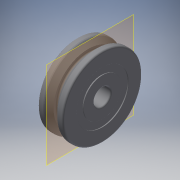
# Autodesk Inventor part: W2RX Bearing
Saved by Autodesk Inventor 2018.3 (Build 223284000, 284)
## iProperties
Category: PARTsolutions
Company: BWC
Created: 2020-02-15
Part Number: W2RX Bearing
Material: Generic
Catalog Web Link: www.cadenas.de
Description: Radial Wheels-Radial Wheels
Vendor: BWC
Document SubType Name: Modeling
Designer: psadmin
Manufacturer: BWC
Mass: 5.93829 g
Surface Area: 30.052 cm^2
Volume: 5.93829 cm^3
Density: 1 g/cm^3
Appearance: PSOLRGB-175-175-175
PSOL_IDENT_0: {$CADENAS_DATA\23d-libs\bwc\madewell\radial_wheels.prj},158 {VTYP=3D},{NB=W2RX},{LINA=W2RX},{NN=Radi
PSOL_IDENT_1: al Wheels},{DATE=05.12.2019 09:46:06},{GEOMDATE=08.11.2014 11:33:08},{VERSION=},{LINEID=30},{WBVAR=M
PSOL_IDENT_2: AT},{WBNUMERIC=}  {NB=W2RX},{LINA=W2RX},{KT=DUMMY},{PN=W2RX},{MAT=RX},{SIZE=2},{D=1.210},{W=0.3830},
PSOL_IDENT_3: {B=0.2510},{VRI=0.5000},{C=0.020},{C1=0.584},{E=0.024},{R=0.028},{R1=0.008},{A=1.3018},{F=0.1250},{R
PSOL_IDENT_4: LN=1500},{RLLBF=337},{ALN=320},{ALLBF=72},{CATEGALG=Radial Wheel, Size 2, Carbon Steel, Sealed},{FEA
PSOL_IDENT_5: TALG=<li style=\" margin-top:0px; margin-bottom:0px; margin-left:0px; margin-right:0px; -qt-block-in
PSOL_IDENT_6: dent:0; text-indent:0px;\"><span style=\" font-size:11pt; font-weight:600;\">General purpose AISI 52
PSOL_IDENT_7: 100 carbon steel</span></li><li style=\" font-size:11pt; font-weight:600;\" style=\" margin-top:0px;
PSOL_IDENT_8: margin-bottom:0px; margin-left:0px; margin-right:0px; -qt-block-indent:0; text-indent:0px;\">Single
PSOL_IDENT_9: row deep-groove ball bearing</li><li style=\" font-size:11pt; font-weight:600;\" style=\" margin-to
PSOL_IDENT_10: p:0px; margin-bottom:0px; margin-left:0px; margin-right:0px; -qt-block-indent:0; text-indent:0px;\">
PSOL_IDENT_11: Precision ground 90° vee inside running surfaces</li><li style=\" font-size:11pt; font-weight:600;\"
PSOL_IDENT_12: style=\" margin-top:0px; margin-bottom:0px; margin-left:0px; margin-right:0px; -qt-block-indent:0;
PSOL_IDENT_13: text-indent:0px;\">Hardened for heavy loads and durability</li><li style=\" font-size:11pt; font-wei
PSOL_IDENT_14: ght:600;\" style=\" margin-top:0px; margin-bottom:0px; margin-left:0px; margin-right:0px; -qt-block-
PSOL_IDENT_15: indent:0; text-indent:0px;\">Seals to protect against contamination</li>},{DESCRALG=<span style=\" f
PSOL_IDENT_16: ont-size:11pt; font-weight:600;\">MadeWell radial wheels are linear guide bearings with single row d
PSOL_IDENT_17: eep-groove ball arrangement with precision ground 90° vee inside surfaces to support loads and provi
PSOL_IDENT_18: de smooth and quiet motion. They are an ideal choice for low cost linear guide bearings in simple li
PSOL_IDENT_19: near guide applications such as doors and windows, museum displays, cabinets, and automation.  Use w
PSOL_IDENT_20: ith DualVee guide track for linear motion. General purpose carbon steel with rubber seals protect ag
PSOL_IDENT_21: ainst small particle contamination. Through bore allows mounting with common bolts and washers. Inte
PSOL_IDENT_22: rnically lubricated for life with general purpose grease.</span>},{RATINGSALG=<span style=\" font-si
PSOL_IDENT_23: ze:11pt; font-weight:600; color:#000000;\">Temperature Range:</span><span style=\" font-size:11pt; c
PSOL_IDENT_24: olor:#000000;\"> -20°C to +100°C</span></p><p style=\" margin-top:0px; margin-bottom:0px; margin-lef
PSOL_IDENT_25: t:0px; margin-right:0px; -qt-block-indent:0; text-indent:0px;\"><span style=\" font-size:11pt; font-
PSOL_IDENT_26: weight:600; color:#000000;\">RoHS Compliant</span>}
NN: Radial Wheels
NT: Radial Wheels
NB: W2RX
NBSYN: $PN.
LINA: W2RX
PN: W2RX
MAT: AISI 52100 Carbon steel
SIZE: 2
D: 1.21
W: 0.383
B: 0.251
VRI: 0.5
RLN: 1500
RLLBF: 337
ALN: 320
ALLBF: 72
SUPPLIER: BWC
ARTICLENO: W2RX
BOMINFO: W2RX
CREATOR: CADENAS GmbH
Title: W2RX
Author: Cadenas PARTsolutions
Comments: Radial Wheels
Autodesk Inventor part; units mm, degrees
sketch "Sketch_1" plane through (0, 0, 0) normal (0, 0, 1) x (1, 0, 0)
  line L0 (4.8641, 0) -> (-4.8641, 0)
  line L1 (-4.8641, 7.3152) -> (-4.8641, 3.6957)
  arc A0 (-4.8641, 3.6957) -> (-4.3561, 3.1877) centre (-4.3561, 3.6957) ccw
  line L2 (-4.3561, 3.1877) -> (4.3561, 3.1877)
  arc A1 (4.3561, 3.1877) -> (4.8641, 3.6957) centre (4.3561, 3.6957) ccw
  line L3 (4.8641, 3.6957) -> (4.8641, 7.3152)
  arc A2 (4.8641, 7.3152) -> (4.7625, 7.4168) centre (4.7625, 7.3152) ccw
  line L4 (4.7625, 7.4168) -> (4.6609, 7.4168)
  arc A3 (4.6609, 7.4168) -> (4.5593, 7.3152) centre (4.6609, 7.3152) ccw
  line L5 (4.5593, 7.3152) -> (4.5593, 7.112)
  line L6 (4.5593, 7.112) -> (4.2545, 7.112)
  line L7 (4.2545, 7.112) -> (4.2545, 10.2616)
  arc A4 (4.3561, 10.3632) -> (4.2545, 10.2616) centre (4.3561, 10.2616) ccw
  line L8 (4.3561, 10.3632) -> (4.5593, 10.3632)
  line L9 (4.5593, 10.3632) -> (4.5593, 10.16)
  arc A5 (4.5593, 10.16) -> (4.6609, 10.0584) centre (4.6609, 10.16) ccw
  line L10 (4.6609, 10.0584) -> (4.7625, 10.0584)
  arc A6 (4.7625, 10.0584) -> (4.8641, 10.16) centre (4.7625, 10.16) ccw
  line L11 (4.8641, 10.16) -> (4.8641, 14.7574)
  arc A7 (4.8641, 14.7574) -> (4.2545, 15.367) centre (4.2545, 14.7574) ccw
  line L12 (4.2545, 15.367) -> (2.8699, 15.367)
  line L13 (2.8699, 15.367) -> (2.523, 15.2233)
  line L14 (2.523, 15.2233) -> (0.7112, 13.4115)
  line L15 (0.7112, 13.4115) -> (0.7112, 12.7)
  arc A8 (-0.7112, 12.7) -> (0.7112, 12.7) centre (0, 12.7) ccw
  line L16 (-0.7112, 12.7) -> (-0.7112, 13.4115)
  line L17 (-0.7112, 13.4115) -> (-2.523, 15.2233)
  line L18 (-2.523, 15.2233) -> (-2.8699, 15.367)
  line L19 (-2.8699, 15.367) -> (-4.2545, 15.367)
  arc A9 (-4.2545, 15.367) -> (-4.8641, 14.7574) centre (-4.2545, 14.7574) ccw
  line L20 (-4.8641, 14.7574) -> (-4.8641, 10.16)
  arc A10 (-4.8641, 10.16) -> (-4.7625, 10.0584) centre (-4.7625, 10.16) ccw
  line L21 (-4.7625, 10.0584) -> (-4.6609, 10.0584)
  arc A11 (-4.6609, 10.0584) -> (-4.5593, 10.16) centre (-4.6609, 10.16) ccw
  line L22 (-4.5593, 10.16) -> (-4.5593, 10.3632)
  line L23 (-4.5593, 10.3632) -> (-4.3561, 10.3632)
  arc A12 (-4.2545, 10.2616) -> (-4.3561, 10.3632) centre (-4.3561, 10.2616) ccw
  line L24 (-4.2545, 10.2616) -> (-4.2545, 7.112)
  line L25 (-4.2545, 7.112) -> (-4.5593, 7.112)
  line L26 (-4.5593, 7.112) -> (-4.5593, 7.3152)
  arc A13 (-4.5593, 7.3152) -> (-4.6609, 7.4168) centre (-4.6609, 7.3152) ccw
  line L27 (-4.6609, 7.4168) -> (-4.7625, 7.4168)
  arc A14 (-4.7625, 7.4168) -> (-4.8641, 7.3152) centre (-4.7625, 7.3152) ccw
  constraints: 56 end point, 30 point on circle, 15 centre point
revolve "Revolution1" add sketch "Sketch_1" angle 360 about axis through (4.8641, 0, 0) along (1, 0, 0)
ref_plane "b_XY" through (-4.6609, 3.1877, 0) normal (0, 0, 1) x (1, 0, 0)
ref_plane "b_YZ" through (-4.6609, 3.1877, 0) normal (1, 0, 0) x (0, 1, 0)
ref_plane "b_ZX" through (-4.6609, 3.1877, 0) normal (0, 1, 0) x (0, 0, 1)
ref_plane "b1_XY" through (-4.6609, -3.1877, 0) normal (0, 0, 1) x (1, 0, 0)
ref_plane "b1_YZ" through (-4.6609, -3.1877, 0) normal (1, 0, 0) x (0, 1, 0)
ref_plane "b1_ZX" through (-4.6609, -3.1877, 0) normal (0, 1, 0) x (0, 0, 1)
ref_plane "d_XY" through (-2.4321, 15.367, 0) normal (0, 0, 1) x (1, 0, 0)
ref_plane "d_YZ" through (-2.4321, 15.367, 0) normal (1, 0, 0) x (0, 1, 0)
ref_plane "d_ZX" through (-2.4321, 15.367, 0) normal (0, 1, 0) x (0, 0, 1)
ref_plane "d1_XY" through (-2.4321, -15.367, 0) normal (0, 0, 1) x (1, 0, 0)
ref_plane "d1_YZ" through (-2.4321, -15.367, 0) normal (1, 0, 0) x (0, 1, 0)
ref_plane "d1_ZX" through (-2.4321, -15.367, 0) normal (0, 1, 0) x (0, 0, 1)
ref_plane "vri_XY" through (0, 12.7, 0) normal (0, 0, 1) x (1, 0, 0)
ref_plane "vri_YZ" through (0, 12.7, 0) normal (1, 0, 0) x (0, 1, 0)
ref_plane "vri_ZX" through (0, 12.7, 0) normal (0, 1, 0) x (0, 0, 1)
ref_plane "vri1_XY" through (4.8641, 0, 0) normal (0, 0, 1) x (1, 0, 0)
ref_plane "vri1_YZ" through (4.8641, 0, 0) normal (1, 0, 0) x (0, 1, 0)
ref_plane "vri1_ZX" through (4.8641, 0, 0) normal (0, 1, 0) x (0, 0, 1)
ref_plane "w_XY" through (-4.8641, 12.7, 0) normal (0, 0, 1) x (1, 0, 0)
ref_plane "w_YZ" through (-4.8641, 12.7, 0) normal (1, 0, 0) x (0, 1, 0)
ref_plane "w_ZX" through (-4.8641, 12.7, 0) normal (0, 1, 0) x (0, 0, 1)
ref_plane "w1_XY" through (4.8641, 12.7, 0) normal (0, 0, 1) x (1, 0, 0)
ref_plane "w1_YZ" through (4.8641, 12.7, 0) normal (1, 0, 0) x (0, 1, 0)
ref_plane "w1_ZX" through (4.8641, 12.7, 0) normal (0, 1, 0) x (0, 0, 1)
ref_plane "wheel_XY" through (4.8641, 0, 0) normal (1, 0, 0) x (0, 0, -1)
ref_plane "wheel_YZ" through (4.8641, 0, 0) normal (0, 0, -1) x (0, 1, 0)
ref_plane "wheel_ZX" through (4.8641, 0, 0) normal (0, 1, 0) x (1, 0, 0)
ref_plane "Work Plane28" through (0, 0, 0) normal (1, 0, 0) x (0, 0, -1)
body "Solid1"
